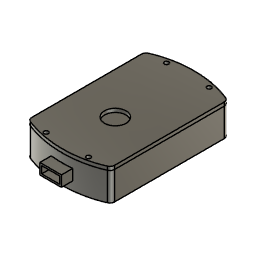
Malla (Autodesk Fusion 360 archive; units mm, degrees)
design "CASE2"
Autodesk Fusion 360 part; units mm, degrees
note: some values were not read from the file. Chosen so that the rebuilt part matches the saved one: where a step ends; which pieces of a blend or face edit are solid. Set by a fixed rule: which face or edge a step refers to; which sketch regions a step uses.
sketch "Boceto1" plane through (0, 0, 0) normal (0, 0, 1) x (1, 0, 0)
  circle A0 centre (-5.9, 16.8256) radius 0.6
  line L0 (10.4, -15.2481) -> (-10.4, -15.2481)
  line L1 (-10.4, 15.5519) -> (-4.2071, 15.5519)
  circle A1 centre (5.9, 16.8256) radius 0.6
  spline S0 degree 3 poles (10.7171, -16.1976) (9.0911, -16.9299) (7.3492, -17.4466) (3.7858, -18.1418) (1.8989, -18.3158) (-4.1389, -18.2732) (-7.7725, -17.3263) (-10.6417, -16.2266) knots -1.732785 -1.732785 -1.732785 -1.732785 -1.337909 -1.337909 -0.921833 -0.921833 0 0 0 0
  line L2 (4.1929, 15.5519) -> (10.4, 15.5519)
  circle A2 centre (0, -16.6178) radius 0.6 construction
  arc A3 (10.7171, -16.1976) -> (11.5, -15.0181) centre (10.22, -15.0181) ccw
  arc A4 (-11.5, -15.0181) -> (-10.6417, -16.2266) centre (-10.22, -15.0181) ccw
  line L3 (10.4, 15.5519) -> (10.4, -15.2481)
  line L4 (11.5, -15.0181) -> (11.4989, 15.4432)
  line L5 (-11.5011, 15.4432) -> (-11.5, -15.0181)
  line L6 (-10.4, -15.2481) -> (-10.4, 15.5519)
  line L7 (4.1929, 15.5519) -> (-4.2071, 15.5519)
  spline S1 degree 3 poles (-10.7181, 16.6227) (-9.0922, 17.355) (-7.3503, 17.8717) (-3.7869, 18.5669) (-1.9, 18.7409) (4.1378, 18.6983) (7.7714, 17.7514) (10.6407, 16.6517) knots -1.732785 -1.732785 -1.732785 -1.732785 -1.337909 -1.337909 -0.921833 -0.921833 0 0 0 0
  arc A5 (11.4989, 15.4432) -> (10.6407, 16.6517) centre (10.2189, 15.4432) ccw
  arc A6 (-10.7181, 16.6227) -> (-11.5011, 15.4432) centre (-10.2211, 15.4432) ccw
  line L8 (-5.9, 16.8256) -> (0, -16.6178) construction
  line L9 (0, -16.6178) -> (-5.9, -16.6178) construction
  line L10 (-5.9, 16.8256) -> (-5.9, -16.6178) construction
  line L11 (0, -16.6178) -> (5.9, 16.8256) construction
  line L12 (5.9, 16.8256) -> (5.9, -16.6178) construction
  line L13 (5.9, -16.6178) -> (0, -16.6178) construction
  circle A7 centre (-5.9, -16.6178) radius 0.6
  circle A8 centre (5.9, -16.6178) radius 0.6
  point P0 (10.3989, 15.6732)
  point P1 (-10.4011, 15.6732)
  dimension "d50" = 1.2
  dimension "d51" = 1.2
  constraint coincident L5.start A6.end
  constraint coincident L4.end A5.start
  constraint coincident A0.centre L8.start
  constraint coincident A2.centre L8.end
  constraint horizontal L9
  constraint perpendicular L9 L10
  constraint coincident A1.centre L11.end
  constraint perpendicular L0 L12
  constraint perpendicular L12 L13
  constraint coincident L9.end L10.end
  constraint coincident L12.end L13.start
  measures "d50" diameter of A7
  measures "d51" diameter of A8
extrude "Extruir1" add sketch "Boceto1" along normal blind 5.6 makes body 1
sketch "Boceto3" plane through (0, 0, 0) normal (0, 0, 1) x (1, 0, 0)
  spline S0 degree 3 poles (-10.7181, 16.6227) (-9.0922, 17.355) (-7.3503, 17.8717) (-3.7869, 18.5669) (-1.9, 18.7409) (4.1378, 18.6983) (7.7714, 17.7514) (10.6407, 16.6517) knots -1.732785 -1.732785 -1.732785 -1.732785 -1.337909 -1.337909 -0.921833 -0.921833 0 0 0 0
  line L0 (-11.5011, 15.4432) -> (-11.5, -15.0181)
  line L1 (11.5, -15.0181) -> (11.4989, 15.4432)
  spline S1 degree 3 poles (10.7171, -16.1976) (9.0911, -16.9299) (7.3492, -17.4466) (3.7858, -18.1418) (1.8989, -18.3158) (-4.1389, -18.2732) (-7.7725, -17.3263) (-10.6417, -16.2266) knots -1.732785 -1.732785 -1.732785 -1.732785 -1.337909 -1.337909 -0.921833 -0.921833 0 0 0 0
  arc A0 (-11.5, -15.0181) -> (-10.6417, -16.2266) centre (-10.22, -15.0181) ccw
  arc A1 (10.7171, -16.1976) -> (11.5, -15.0181) centre (10.22, -15.0181) ccw
  arc A2 (11.4989, 15.4432) -> (10.6407, 16.6517) centre (10.2189, 15.4432) ccw
  arc A3 (-10.7181, 16.6227) -> (-11.5011, 15.4432) centre (-10.2211, 15.4432) ccw
  point P0 (10.3989, 15.6732)
  point P1 (-10.4011, 15.6732)
  constraint coincident L0.start A3.end
  constraint coincident L1.end A2.start
extrude "Extruir2" add sketch "Boceto3" against normal blind 2.2 bodies 1
sketch "Boceto4" plane through (0, 0, 5.6) normal (0, 0, 1) x (-1, 0, 0)
  circle A0 centre (-5.9, -16.8256) radius 0.6
  circle A1 centre (5.9, -16.8256) radius 0.6
  line L0 (10.4, -15.5519) -> (-10.4, -15.5519)
  line L1 (-10.4, -15.5519) -> (-10.4, 15.2481)
  line L2 (-10.4, 15.2481) -> (10.4, 15.2481)
  line L3 (10.4, 15.2481) -> (10.4, -15.5519)
  arc A2 (-10.7171, 16.1976) -> (-11.5, 15.0181) centre (-10.22, 15.0181) ccw
  line L4 (-11.5, 15.0181) -> (-11.4989, -15.4432)
  line L5 (11.5011, -15.4432) -> (11.5, 15.0181)
  arc A3 (11.5, 15.0181) -> (10.6417, 16.2266) centre (10.22, 15.0181) ccw
  spline S0 degree 3 poles (10.6417, 16.2266) (7.7725, 17.3263) (4.1389, 18.2732) (-1.8989, 18.3158) (-3.7858, 18.1418) (-7.3492, 17.4466) (-9.0911, 16.9299) (-10.7171, 16.1976) knots 0 0 0 0 0.921833 0.921833 1.337909 1.337909 1.732785 1.732785 1.732785 1.732785
  line L6 (0, 16.6178) -> (0, 18.3024) construction
  line L7 (0, 18.3024) -> (0, 21.3024) construction
  line L8 (0, 21.3024) -> (5.4941, 21.3024) construction
  line L9 (0, -15.5519) -> (0, -18.7275) construction
  line L10 (0, -18.7275) -> (0, -21.7275) construction
  line L11 (0, -21.7275) -> (4.3514, -21.7275) construction
  arc A4 (-11.4989, -15.4432) -> (-10.6407, -16.6517) centre (-10.2189, -15.4432) ccw
  spline S1 degree 3 poles (-10.6407, -16.6517) (-7.7714, -17.7514) (-4.1378, -18.6983) (1.9, -18.7409) (3.7869, -18.5669) (7.3503, -17.8717) (9.0922, -17.355) (10.7181, -16.6227) knots 0 0 0 0 0.921833 0.921833 1.337909 1.337909 1.732785 1.732785 1.732785 1.732785
  arc A5 (10.7181, -16.6227) -> (11.5011, -15.4432) centre (10.2211, -15.4432) ccw
  line L12 (5.9, -16.8256) -> (0, 16.6178) construction
  line L13 (5.9, 16.6178) -> (0, 16.6178) construction
  line L14 (5.9, 16.6178) -> (5.9, -16.8256) construction
  line L15 (0, 16.6178) -> (-5.9, -16.8256) construction
  line L16 (-5.9, -16.8256) -> (-5.9012, 16.6178) construction
  line L17 (-5.9012, 16.6178) -> (0, 16.6178) construction
  circle A6 centre (5.9, 16.6178) radius 0.6
  circle A7 centre (-5.9012, 16.6178) radius 0.6
  circle A8 centre (-5.9, 16.6178) radius 0.6
  circle A9 centre (5.9, 16.6178) radius 0.6
  dimension "d6" = 3
  dimension "d7" = 3
  dimension "d45" = 1.2
  dimension "d46" = 1.2
  constraint coincident S0 L6.end
  constraint vertical L6
  constraint parallel L6 L7
  constraint perpendicular L7 L8
  constraint midpoint L0 L9.start
  constraint perpendicular L0 L9
  constraint perpendicular L0 L10
  constraint perpendicular L10 L11
  constraint coincident A1.centre L12.start
  constraint perpendicular L6 L13
  constraint perpendicular L0 L14
  constraint coincident A0.centre L15.end
  constraint parallel L4 L16
  constraint parallel L13 L17
  constraint coincident L13.start L14.start
  constraint coincident L16.end L17.start
  constraint coincident L9.end S1
  measures "d6" distance of L6.end L7.end
  measures "d7" distance of L9.end L10.end
  measures "d45" diameter of A6
  measures "d46" diameter of A7
ref_plane "PlanoDeObra1" through (-2.747, -21.3024, 5.6) normal (0, 1, 0) x (-1, 0, 0)
ref_plane "PlanoDeObra2" through (-2.1757, 21.7275, 5.6) normal (0, 1, 0) x (-1, 0, 0)
sketch "Boceto5" plane through (0, -21.3024, 0) normal (0, 1, 0) x (1, 0, 0)
  line L0 (10.7171, 2.2) -> (10.7171, -5.6)
  line L1 (-10.6417, -5.6) -> (10.7171, -5.6)
  line L2 (-10.6417, -5.6) -> (-10.6417, 2.2)
  line L3 (10.7171, 2.2) -> (-10.6417, 2.2)
  line L4 (-10.6417, -5.6) -> (-2.4623, -2.613) construction
  line L5 (2.5377, -1.7) -> (2.5377, -2.7)
  line L6 (2.5377, -0.7) -> (-2.4623, -0.7)
  line L7 (-2.4623, -0.7) -> (-2.4623, -2.7)
  line L8 (-2.4623, -2.7) -> (2.5377, -2.7)
  line L9 (-10.6417, 2.2) -> (-2.4623, -0.787) construction
  line L10 (2.5377, -2.613) -> (10.7171, -5.6) construction
  line L11 (2.5377, -1.7) -> (2.5377, -0.7)
  line L12 (2.5377, -0.7) -> (3.0377, -0.2) construction
  line L13 (2.5377, -0.7) -> (3.9519, -0.7) construction
  line L14 (3.0377, -0.2) -> (3.0377, -3.2)
  line L15 (3.0377, -0.2) -> (-2.9623, -0.2)
  line L16 (-2.9623, -0.2) -> (-2.9623, -3.2)
  line L17 (-2.9623, -3.2) -> (3.0377, -3.2)
  dimension "d63" = 1
  dimension "d64" = 1
  dimension "d65" = 5
  dimension "d66" = 2
  dimension "d67" = 45
  dimension "d68" = 0.7071
  dimension "d69" = 3
  dimension "d70" = 6
  dimension "d71" = 3
  constraint coincident L1.start L2.start
  constraint coincident L2.end L3.end
  constraint coincident L0.end L1.end
  constraint coincident L5 L10.start
  constraint collinear L9 L10
  constraint coincident L7 L9.end
  constraint coincident L7 L4.end
  constraint perpendicular L6 L11
  constraint horizontal L13
  constraint vertical L14
  constraint perpendicular L14 L15
  constraint perpendicular L15 L16
  measures "d63" distance of L5.start L5.end
  measures "d64" distance of L5.start L6.start
  measures "d65" distance of L6.start L6.end
  measures "d66" distance of L6.end L7.end
  measures "d67" angle of L12 L13
  measures "d68" distance of L6.start L12.end
  measures "d69" distance of L12.end L14.end
  measures "d70" distance of L12.end L15.end
  measures "d71" distance of L15.end L16.end
extrude "Extruir3" add sketch "Boceto5" along normal up to near side of body 1 contours L14 L15 L16 L17 bodies 1
sketch "Boceto6" plane through (0, 21.7275, 0) normal (0, 1, 0) x (1, 0, 0)
  line L0 (-10.7181, 2.2) -> (-10.7181, -5.6)
  line L1 (10.6407, -5.6) -> (-10.7181, -5.6)
  line L2 (10.6407, -5.6) -> (10.6407, 2.2)
  line L3 (-10.7181, 2.2) -> (10.6407, 2.2)
  line L4 (1.7637, -2.3582) -> (-1.7363, -1.0801) construction
  line L5 (10.6407, 2.2) -> (-1.7363, -2.3199) construction
  line L6 (-0.0387, -1.7) -> (-1.2887, -1.7) construction
  line L7 (-1.2887, -1.7) -> (-1.2887, -0.7)
  line L8 (-1.2887, -1.7) -> (-1.2887, -2.7) construction
  line L9 (-1.2887, -2.7) -> (1.2113, -2.7)
  line L10 (1.2113, -2.7) -> (1.2113, -0.7)
  line L11 (1.2113, -0.7) -> (-1.2887, -0.7)
  line L12 (-1.2887, -1.7) -> (-1.2887, -2.7)
  line L13 (-1.2887, -0.7) -> (-1.7887, -0.7) construction
  line L14 (-1.2887, -0.7) -> (-1.2887, -0.2) construction
  line L15 (-1.2887, -0.2) -> (-1.7887, -0.2) construction
  line L16 (-1.7887, -0.2) -> (-1.7887, -0.7) construction
  line L17 (-1.7887, -0.2) -> (-1.7887, -3.2)
  line L18 (-1.7887, -0.2) -> (1.7113, -0.2)
  line L19 (1.7113, -0.2) -> (1.7113, -3.2)
  line L20 (1.7113, -3.2) -> (-1.7887, -3.2)
  dimension "d103" = 1.25
  dimension "d104" = 1
  dimension "d105" = 1
  dimension "d106" = 2.5
  dimension "d107" = 2
  dimension "d112" = 0.5
  dimension "d113" = 0.5
  dimension "d114" = 3
  dimension "d115" = 3.5
  dimension "d116" = 3
  constraint coincident L2.end L3.end
  constraint perpendicular L0 L6
  constraint perpendicular L6 L7
  constraint perpendicular L6 L8
  constraint perpendicular L8 L9
  constraint perpendicular L9 L10
  constraint coincident L5 L6.start
  constraint perpendicular L7 L13
  constraint perpendicular L11 L14
  constraint perpendicular L14 L15
  constraint perpendicular L13 L16
  constraint perpendicular L15 L17
  constraint perpendicular L16 L18
  constraint perpendicular L18 L19
  measures "d103" distance of L6.start L6.end
  measures "d104" distance of L6.end L7.end
  measures "d105" distance of L6.end L8.end
  measures "d106" distance of L8.end L9.end
  measures "d107" distance of L9.end L10.end
  measures "d112" distance of L7.end L13.end
  measures "d113" distance of L7.end L14.end
  measures "d114" distance of L15.end L17.end
  measures "d115" distance of L15.end L18.end
  measures "d116" distance of L18.end L19.end
extrude "Extruir4" add sketch "Boceto6" against normal up to surface (6.1755 mm away) contours L17 L18 L19 L20 bodies 1
sketch "Boceto7" plane through (0, 0, -2.2) normal (0, 0, -1) x (1, 0, 0)
  line L0 (11.4989, -15.4432) -> (11.5, 15.0181)
  arc A0 (11.5, 15.0181) -> (10.7171, 16.1976) centre (10.22, 15.0181) ccw
  spline S0 degree 3 poles (10.7171, 16.1976) (9.0911, 16.9299) (7.3492, 17.4466) (3.7858, 18.1418) (1.8989, 18.3158) (-4.1389, 18.2732) (-7.7725, 17.3263) (-10.6417, 16.2266) knots -1.732785 -1.732785 -1.732785 -1.732785 -1.337909 -1.337909 -0.921833 -0.921833 0 0 0 0
  arc A1 (-10.6417, 16.2266) -> (-11.5, 15.0181) centre (-10.22, 15.0181) ccw
  line L1 (-11.5, 15.0181) -> (-11.5011, -15.4432)
  arc A2 (-5.775, -6.6) -> (-5.775, -15) centre (-5.775, -10.8) ccw
  line L2 (5.775, 4.2) -> (-5.775, 4.2)
  arc A3 (5.775, -4.2) -> (5.775, 4.2) centre (5.775, 0) ccw
  arc A4 (5.775, -15) -> (5.775, -6.6) centre (5.775, -10.8) ccw
  line L3 (5.775, 15) -> (-5.775, 15)
  arc A5 (5.775, 6.6) -> (5.775, 15) centre (5.775, 10.8) ccw
  line L4 (-5.775, -15) -> (5.775, -15)
  arc A6 (-5.775, 4.2) -> (-5.775, -4.2) centre (-5.775, 0) ccw
  line L5 (-5.775, 6.6) -> (5.775, 6.6)
  arc A7 (-5.775, 15) -> (-5.775, 6.6) centre (-5.775, 10.8) ccw
  line L6 (-5.775, -4.2) -> (5.775, -4.2)
  line L7 (5.775, -6.6) -> (-5.775, -6.6)
  arc A8 (-11.5011, -15.4432) -> (-10.7181, -16.6227) centre (-10.2211, -15.4432) ccw
  spline S1 degree 3 poles (-10.7181, -16.6227) (-9.0922, -17.355) (-7.3503, -17.8717) (-3.7869, -18.5669) (-1.9, -18.7409) (4.1378, -18.6983) (7.7714, -17.7514) (10.6407, -16.6517) knots -1.732785 -1.732785 -1.732785 -1.732785 -1.337909 -1.337909 -0.921833 -0.921833 0 0 0 0
  arc A9 (10.6407, -16.6517) -> (11.4989, -15.4432) centre (10.2189, -15.4432) ccw
sketch "Boceto8" plane through (0, 0, 0) normal (0, 0, 1) x (-1, 0, 0)
  line L0 (10.4, -15.5519) -> (10.4, 15.2481)
  line L1 (10.4, 15.2481) -> (-10.4, 15.2481)
  line L2 (-10.4, 15.2481) -> (-10.4, -15.5519)
  line L3 (-10.4, -15.5519) -> (10.4, -15.5519)
  arc A0 (-1, 1.0002) -> (-1, -0.9998) centre (-1, 0.0002) ccw
  line L4 (3, 1.0002) -> (3, 1.0002)
  arc A1 (-1, 1.0002) -> (-1, -0.9998) centre (-1, 0.0002) ccw
  line L5 (-1, 11.7998) -> (3, 11.7998)
  line L6 (3, -11.7997) -> (-1, -11.7997)
  arc A2 (-1, -9.7997) -> (-1, -11.7997) centre (-1, -10.7997) ccw
  arc A3 (3, 9.7998) -> (3, 11.7998) centre (3, 10.7998) ccw
  arc A4 (3, -0.9998) -> (3, 1.0002) centre (3, 0.0002) ccw
  line L7 (-1, -11.7997) -> (3, -11.7997)
  line L8 (3, 9.7998) -> (-1, 9.7998)
  line L9 (-1, -0.9998) -> (3, -0.9998)
  arc A5 (3, -11.7997) -> (3, -9.7997) centre (3, -10.7997) ccw
  line L10 (3, -0.9998) -> (-1, -0.9998)
  line L11 (3, -9.7997) -> (-1, -9.7997)
  arc A6 (-1, 11.7998) -> (-1, 9.7998) centre (-1, 10.7998) ccw
  arc A7 (3, -0.9998) -> (3, 1.0002) centre (3, 0.0002) ccw
  arc A8 (3, -11.7997) -> (3, -9.7997) centre (3, -10.7997) ccw
  line L12 (-1, 1.0002) -> (3, 1.0002)
  arc A9 (-1, -9.7997) -> (-1, -11.7997) centre (-1, -10.7997) ccw
  line L13 (-1, 0.8945) -> (-1, 0.8945)
  line L14 (-1, 1.8945) -> (-1, 1.8945)
  line L15 (3, 1.8945) -> (3, 1.8945)
  line L16 (-1, -9.7997) -> (3, -9.7997)
  line L17 (3, 0.8945) -> (3, 0.8945)
extrude "Extruir5" cut sketch "Boceto8" against normal blind 1 contours A0 A1 A4 L9 L10 A7 L12 | L5 A3 L8 A6 | L6 A2 L7 A5 L11 A8 A9 L16 bodies 1
extrude "Extruir6" cut sketch "Boceto7" against normal blind 1.2 contours A2 A4 L4 L7 | L2 A3 A6 L6 | L3 A5 L5 A7 bodies 1
ref_plane "PlanoDeObra3" through (-0.0005, 0.2126, 5.6) normal (0, 0, 1) x (1, 0, 0)
sketch "Boceto9" plane through (0, 0, 5.6) normal (0, 0, 1) x (1, 0, 0)
  arc A0 (-10.7181, 16.6227) -> (-11.5011, 15.4432) centre (-10.2211, 15.4432) ccw
  arc A1 (11.4989, 15.4432) -> (10.6407, 16.6517) centre (10.2189, 15.4432) ccw
  line L0 (-10.4, 15.5519) -> (-4.2071, 15.5519)
  line L1 (-11.5011, 15.4432) -> (-11.5, -15.0181)
  circle A2 centre (-5.9, 16.8256) radius 0.6
  arc A3 (10.7171, -16.1976) -> (11.5, -15.0181) centre (10.22, -15.0181) ccw
  line L2 (11.5, -15.0181) -> (11.4989, 15.4432)
  spline S0 degree 3 poles (-10.7181, 16.6227) (-9.0922, 17.355) (-7.3503, 17.8717) (-3.7869, 18.5669) (-1.9, 18.7409) (4.1378, 18.6983) (7.7714, 17.7514) (10.6407, 16.6517) knots -1.732785 -1.732785 -1.732785 -1.732785 -1.337909 -1.337909 -0.921833 -0.921833 0 0 0 0
  line L3 (10.4, 15.5519) -> (10.4, -15.2481)
  line L4 (4.1929, 15.5519) -> (10.4, 15.5519)
  line L5 (-10.4, -15.2481) -> (-10.4, 15.5519)
  line L6 (4.1929, 15.5519) -> (-4.2071, 15.5519)
  spline S1 degree 3 poles (10.7171, -16.1976) (9.0911, -16.9299) (7.3492, -17.4466) (3.7858, -18.1418) (1.8989, -18.3158) (-4.1389, -18.2732) (-7.7725, -17.3263) (-10.6417, -16.2266) knots -1.732785 -1.732785 -1.732785 -1.732785 -1.337909 -1.337909 -0.921833 -0.921833 0 0 0 0
  arc A4 (-11.5, -15.0181) -> (-10.6417, -16.2266) centre (-10.22, -15.0181) ccw
  line L7 (10.4, -15.2481) -> (-10.4, -15.2481)
  circle A5 centre (5.9, 16.8256) radius 0.6
  line L8 (0, -16.6178) -> (-5.9, 16.8256) construction
  line L9 (0, -16.6178) -> (5.9, 16.8256) construction
  line L10 (5.9, 16.8256) -> (5.9, -16.6178) construction
  line L11 (5.9, -16.6178) -> (0, -16.6178) construction
  circle A6 centre (5.9, -16.6178) radius 0.6
  line L12 (-5.9, 16.8256) -> (-5.8943, 16.2256)
  line L13 (-5.9, 16.8256) -> (-5.8943, -17.1357) construction
  line L14 (0, -16.6178) -> (-5.8943, -16.6188) construction
  circle A7 centre (-5.8943, -16.6188) radius 0.6
  point P0 (10.3989, 15.6732)
  point P1 (-10.4011, 15.6732)
  dimension "d48" = 1.2
  dimension "d49" = 1.2
  constraint coincident A0.end L1.start
  constraint coincident A1.start L2.end
  constraint coincident A2.centre L8.end
  constraint coincident A5.centre L9.end
  constraint perpendicular L7 L10
  constraint perpendicular L10 L11
  constraint coincident L10.end L11.start
  constraint coincident A2 L12.end
  constraint coincident L13 L14.end
  constraint perpendicular L13 L14
  constraint coincident L14.end A7.centre
  measures "d48" diameter of A6
  measures "d49" diameter of A7
extrude "Extruir7" add sketch "Boceto9" along normal blind 1 separate body contours A0 A1 L1 A3 L2 S0 S1 A4 | L0 L3 L4 L5 L6 L7 makes body 2
sketch "Boceto10" plane through (0, 0, 6.6) normal (0, 0, 1) x (-1, 0, 0)
  circle A0 centre (-5.9, -16.8256) radius 0.6
  circle A1 centre (5.9, -16.8256) radius 0.6
  arc A2 (10.7181, -16.6227) -> (11.5011, -15.4432) centre (10.2211, -15.4432) ccw
  line L0 (11.5011, -15.4432) -> (11.5, 15.0181)
  arc A3 (11.5, 15.0181) -> (10.6417, 16.2266) centre (10.22, 15.0181) ccw
  spline S0 degree 3 poles (10.6417, 16.2266) (7.7725, 17.3263) (4.1389, 18.2732) (-1.8989, 18.3158) (-3.7858, 18.1418) (-7.3492, 17.4466) (-9.0911, 16.9299) (-10.7171, 16.1976) knots 0 0 0 0 0.921833 0.921833 1.337909 1.337909 1.732785 1.732785 1.732785 1.732785
  arc A4 (-10.7171, 16.1976) -> (-11.5, 15.0181) centre (-10.22, 15.0181) ccw
  line L1 (-11.5, 15.0181) -> (-11.4989, -15.4432)
  arc A5 (-11.4989, -15.4432) -> (-10.6407, -16.6517) centre (-10.2189, -15.4432) ccw
  spline S1 degree 3 poles (-10.6407, -16.6517) (-7.7714, -17.7514) (-4.1378, -18.6983) (1.9, -18.7409) (3.7869, -18.5669) (7.3503, -17.8717) (9.0922, -17.355) (10.7181, -16.6227) knots 0 0 0 0 0.921833 0.921833 1.337909 1.337909 1.732785 1.732785 1.732785 1.732785
  line L2 (0, 16.6178) -> (0, 3.3178) construction
  circle A6 centre (0, 3.3178) radius 3
  circle A7 centre (-5.9, 16.6178) radius 0.6
  circle A8 centre (5.8943, 16.6188) radius 0.6
  dimension "d43" = 13.3
  dimension "d44" = 6
  constraint vertical L2
  constraint coincident L2.end A6.centre
  measures "d43" distance of L2.start L2.end
  measures "d44" diameter of A6
extrude "Extruir8" cut sketch "Boceto10" against normal through all contours A6 bodies 2
delete_face "SuprimirCaras1" 1 faces at (-1.6499, -18.2413, 1.5889) on bodies 1
delete_face "SuprimirCaras2" 1 faces at (0.8037, 18.7097, 1.5889) on bodies 1
equation "d68 = ( sqrt(2) ) * 0.5 mm"
equation "d103 = ( 2.5 / 2 ) * 1 mm"
named bodies: "Case", "Tapa"
